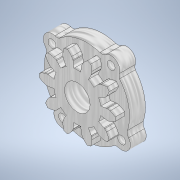
# Autodesk Inventor part: ｍ2歯数10ギア改二
Saved by Autodesk Inventor 2020.2 (Build 242310000, 310)
## iProperties
Created: 2019-11-09
Part Number: ｍ2歯数10ギア改二
Material: アルミニウム 7075
Document SubType Name: Modeling
Designer: aoyam
Density: 2.81 g/cm^3
Appearance: サテン - ブラシ仕上げ 重厚
Author: aoyam
Autodesk Inventor part; units mm, degrees
ref_plane "YZ Plane" through (0, 0, 0) normal (1, 0, 0) x (0, 1, 0)
ref_plane "XZ Plane" through (0, 0, 0) normal (0, 1, 0) x (-1, 0, 0)
ref_plane "XY Plane" through (0, 0, 0) normal (0, 0, 1) x (1, 0, 0)
sketch "スケッチ1" plane through (0, 0, 0) normal (0, 0, 1) x (1, 0, 0)
  arc A0 (-6.7711, 4.8044) -> (-6.8414, 4.5719) centre (-5.6655, 4.3429) ccw
  arc A1 (-6.3619, 5.5344) -> (-6.7711, 4.8044) centre (-3.6713, 3.5464) ccw
  arc A2 (-5.0279, 6.8503) -> (-6.3619, 5.5344) centre (-1.5449, 1.9856) ccw
  arc A3 (-9.5045, 4.5719) -> (-9.5748, 4.8044) centre (-10.6804, 4.3429) ccw
  arc A4 (-9.5748, 4.8044) -> (-9.984, 5.5344) centre (-12.6746, 3.5464) ccw
  arc A5 (-9.984, 5.5344) -> (-11.318, 6.8503) centre (-14.801, 1.9856) ccw
  arc A6 (-7.1102, 2.6941) -> (-9.2357, 2.6941) centre (-8.1729, -4.7302) ccw
  arc A7 (-11.318, 6.8503) -> (-12.4354, 6.4873) centre (-8.1729, -4.7302) ccw
  line L0 (-7.1102, 2.6941) -> (-6.8414, 4.5719)
  line L1 (-9.2357, 2.6941) -> (-9.5045, 4.5719)
  line L2 (-22.1729, -4.7302) -> (5.8271, -4.7302)
  line L3 (-8.1729, -18.7302) -> (-8.1729, 9.2698)
  arc A8 (-11.6771, 1.9009) -> (-13.3966, 0.6516) centre (-8.1729, -4.7302) ccw
  line L4 (-11.6771, 1.9009) -> (-12.5634, 3.578)
  line L5 (-13.3966, 0.6516) -> (-14.7178, 2.0127)
  arc A9 (-14.7178, 2.0127) -> (-14.9114, 2.1595) centre (-15.5346, 1.1363) ccw
  arc A10 (-12.4354, 6.4873) -> (-12.7411, 4.6385) centre (-6.7582, 4.5989) ccw
  arc A11 (-14.9114, 2.1595) -> (-15.6715, 2.5095) centre (-16.6797, -0.6803) ccw
  arc A12 (-15.6715, 2.5095) -> (-17.5242, 2.7901) centre (-17.4826, -3.1929) ccw
  arc A13 (-17.5242, 2.7901) -> (-18.2148, 1.8395) centre (-8.1729, -4.7302) ccw
  arc A14 (-12.6431, 3.8075) -> (-12.5634, 3.578) centre (-11.4774, 4.084) ccw
  arc A15 (-12.7411, 4.6385) -> (-12.6431, 3.8075) centre (-9.3959, 4.6117) ccw
  arc A16 (-14.9055, -1.4252) -> (-15.5623, -3.4467) centre (-8.1729, -4.7302) ccw
  line L6 (-14.9055, -1.4252) -> (-16.6083, -0.5893)
  line L7 (-15.5623, -3.4467) -> (-17.4312, -3.122)
  arc A17 (-17.4312, -3.122) -> (-17.6741, -3.1171) centre (-17.5768, -4.3112) ccw
  arc A18 (-18.2148, 1.8395) -> (-17.3755, 0.1642) centre (-12.5119, 3.6488) ccw
  arc A19 (-17.6741, -3.1171) -> (-18.4948, -3.2807) centre (-17.4355, -6.4539) ccw
  arc A20 (-18.4948, -3.2807) -> (-20.1586, -4.1427) centre (-16.6083, -8.9586) ccw
  arc A21 (-20.1586, -4.1427) -> (-20.1586, -5.3177) centre (-8.1729, -4.7302) ccw
  arc A22 (-16.8077, -0.4506) -> (-16.6083, -0.5893) centre (-16.0272, 0.4583) ccw
  arc A23 (-17.3755, 0.1642) -> (-16.8077, -0.4506) centre (-14.6534, 2.1087) ccw
  arc A24 (-15.5623, -6.0137) -> (-14.9055, -8.0351) centre (-8.1729, -4.7302) ccw
  line L8 (-15.5623, -6.0137) -> (-17.4312, -6.3384)
  line L9 (-14.9055, -8.0351) -> (-16.6083, -8.871)
  arc A25 (-16.6083, -8.871) -> (-16.8077, -9.0098) centre (-16.0272, -9.9187) ccw
  arc A26 (-20.1586, -5.3177) -> (-18.4948, -6.1797) centre (-16.6083, -0.5018) ccw
  arc A27 (-16.8077, -9.0098) -> (-17.3755, -9.6246) centre (-14.6534, -11.5691) ccw
  arc A28 (-17.3755, -9.6246) -> (-18.2148, -11.2999) centre (-12.5119, -13.1092) ccw
  arc A29 (-18.2148, -11.2999) -> (-17.5242, -12.2504) centre (-8.1729, -4.7302) ccw
  arc A30 (-17.6741, -6.3433) -> (-17.4312, -6.3384) centre (-17.5768, -5.1492) ccw
  arc A31 (-18.4948, -6.1797) -> (-17.6741, -6.3433) centre (-17.4355, -3.0065) ccw
  arc A32 (-13.3966, -10.1119) -> (-11.6771, -11.3612) centre (-8.1729, -4.7302) ccw
  line L10 (-13.3966, -10.1119) -> (-14.7178, -11.4731)
  line L11 (-11.6771, -11.3612) -> (-12.5634, -13.0384)
  arc A33 (-12.5634, -13.0384) -> (-12.6431, -13.2679) centre (-11.4774, -13.5443) ccw
  arc A34 (-17.5242, -12.2504) -> (-15.6715, -11.9699) centre (-17.4826, -6.2675) ccw
  arc A35 (-12.6431, -13.2679) -> (-12.7411, -14.0989) centre (-9.3959, -14.0721) ccw
  arc A36 (-12.7411, -14.0989) -> (-12.4354, -15.9476) centre (-6.7582, -14.0593) ccw
  arc A37 (-12.4354, -15.9476) -> (-11.318, -16.3107) centre (-8.1729, -4.7302) ccw
  arc A38 (-14.9114, -11.6198) -> (-14.7178, -11.4731) centre (-15.5346, -10.5967) ccw
  arc A39 (-15.6715, -11.9699) -> (-14.9114, -11.6198) centre (-16.6797, -8.7801) ccw
  arc A40 (-9.2357, -12.1545) -> (-7.1102, -12.1545) centre (-8.1729, -4.7302) ccw
  line L12 (-9.2357, -12.1545) -> (-9.5045, -14.0323)
  line L13 (-7.1102, -12.1545) -> (-6.8414, -14.0323)
  arc A41 (-6.8414, -14.0323) -> (-6.7711, -14.2648) centre (-5.6655, -13.8033) ccw
  arc A42 (-11.318, -16.3107) -> (-9.984, -14.9948) centre (-14.801, -11.446) ccw
  arc A43 (-6.7711, -14.2648) -> (-6.3619, -14.9948) centre (-3.6713, -13.0068) ccw
  arc A44 (-6.3619, -14.9948) -> (-5.0279, -16.3107) centre (-1.5449, -11.446) ccw
  arc A45 (-5.0279, -16.3107) -> (-3.9105, -15.9476) centre (-8.1729, -4.7302) ccw
  arc A46 (-9.5748, -14.2648) -> (-9.5045, -14.0323) centre (-10.6804, -13.8033) ccw
  arc A47 (-9.984, -14.9948) -> (-9.5748, -14.2648) centre (-12.6746, -13.0068) ccw
  arc A48 (-4.6688, -11.3612) -> (-2.9493, -10.1119) centre (-8.1729, -4.7302) ccw
  line L14 (-4.6688, -11.3612) -> (-3.7825, -13.0384)
  line L15 (-2.9493, -10.1119) -> (-1.6281, -11.4731)
  arc A49 (-1.6281, -11.4731) -> (-1.4345, -11.6198) centre (-0.8113, -10.5967) ccw
  arc A50 (-3.9105, -15.9476) -> (-3.6048, -14.0989) centre (-9.5877, -14.0593) ccw
  arc A51 (-1.4345, -11.6198) -> (-0.6744, -11.9699) centre (0.3338, -8.7801) ccw
  arc A52 (-0.6744, -11.9699) -> (1.1783, -12.2504) centre (1.1367, -6.2675) ccw
  arc A53 (1.1783, -12.2504) -> (1.8689, -11.2999) centre (-8.1729, -4.7302) ccw
  arc A54 (-3.7028, -13.2679) -> (-3.7825, -13.0384) centre (-4.8685, -13.5443) ccw
  arc A55 (-3.6048, -14.0989) -> (-3.7028, -13.2679) centre (-6.95, -14.0721) ccw
  arc A56 (-1.4404, -8.0351) -> (-0.7836, -6.0137) centre (-8.1729, -4.7302) ccw
  line L16 (-1.4404, -8.0351) -> (0.2624, -8.871)
  line L17 (-0.7836, -6.0137) -> (1.0853, -6.3384)
  arc A57 (1.0853, -6.3384) -> (1.3282, -6.3433) centre (1.2309, -5.1492) ccw
  arc A58 (1.8689, -11.2999) -> (1.0296, -9.6246) centre (-3.834, -13.1092) ccw
  arc A59 (1.3282, -6.3433) -> (2.1489, -6.1797) centre (1.0897, -3.0065) ccw
  arc A60 (2.1489, -6.1797) -> (3.8127, -5.3177) centre (0.2624, -0.5018) ccw
  arc A61 (3.8127, -5.3177) -> (3.8127, -4.1427) centre (-8.1729, -4.7302) ccw
  arc A62 (0.4618, -9.0098) -> (0.2624, -8.871) centre (-0.3187, -9.9187) ccw
  arc A63 (1.0296, -9.6246) -> (0.4618, -9.0098) centre (-1.6925, -11.5691) ccw
  arc A64 (-0.7836, -3.4467) -> (-1.4404, -1.4252) centre (-8.1729, -4.7302) ccw
  line L18 (-0.7836, -3.4467) -> (1.0853, -3.122)
  line L19 (-1.4404, -1.4252) -> (0.2624, -0.5893)
  arc A65 (0.2624, -0.5893) -> (0.4618, -0.4506) centre (-0.3187, 0.4583) ccw
  arc A66 (3.8127, -4.1427) -> (2.1489, -3.2807) centre (0.2624, -8.9586) ccw
  arc A67 (0.4618, -0.4506) -> (1.0296, 0.1642) centre (-1.6925, 2.1087) ccw
  arc A68 (1.0296, 0.1642) -> (1.8689, 1.8395) centre (-3.834, 3.6488) ccw
  arc A69 (1.8689, 1.8395) -> (1.1783, 2.7901) centre (-8.1729, -4.7302) ccw
  arc A70 (1.3282, -3.1171) -> (1.0853, -3.122) centre (1.2309, -4.3112) ccw
  arc A71 (2.1489, -3.2807) -> (1.3282, -3.1171) centre (1.0897, -6.4539) ccw
  arc A72 (-2.9493, 0.6516) -> (-4.6688, 1.9009) centre (-8.1729, -4.7302) ccw
  line L20 (-2.9493, 0.6516) -> (-1.6281, 2.0127)
  line L21 (-4.6688, 1.9009) -> (-3.7825, 3.578)
  arc A73 (-3.7825, 3.578) -> (-3.7028, 3.8075) centre (-4.8685, 4.084) ccw
  arc A74 (1.1783, 2.7901) -> (-0.6744, 2.5095) centre (1.1367, -3.1929) ccw
  arc A75 (-3.7028, 3.8075) -> (-3.6048, 4.6385) centre (-6.95, 4.6117) ccw
  arc A76 (-3.6048, 4.6385) -> (-3.9105, 6.4873) centre (-9.5877, 4.5989) ccw
  arc A77 (-3.9105, 6.4873) -> (-5.0279, 6.8503) centre (-8.1729, -4.7302) ccw
  arc A78 (-1.4345, 2.1595) -> (-1.6281, 2.0127) centre (-0.8113, 1.1363) ccw
  arc A79 (-0.6744, 2.5095) -> (-1.4345, 2.1595) centre (0.3338, -0.6803) ccw
  circle A80 centre (-8.1729, -4.7302) radius 2.5
  circle A81 centre (-8.1729, -4.7302) radius 4.025
  circle A82 centre (-8.1729, -4.7302) radius 12 construction
  circle A83 centre (-19.1875, 2.9441) radius 1.25
  arc A84 (-18.2949, 5.5452) -> (-21.3532, 1.2493) centre (-19.1875, 2.9441) ccw
  arc A85 (-18.2949, 5.5452) -> (-16.8738, 5.5919) centre (-17.6457, 7.4369) ccw
  arc A86 (-21.0243, -0.5958) -> (-21.3532, 1.2493) centre (-22.9282, 0.0167) ccw
  arc A87 (-18.4484, -14.8521) -> (-14.1525, -17.9104) centre (-15.8473, -15.7447) ccw
  circle A88 centre (-15.8473, -15.7447) radius 1.25
  arc A89 (-12.3074, -17.5815) -> (-14.1525, -17.9104) centre (-12.9199, -19.4854) ccw
  arc A90 (-18.4484, -14.8521) -> (-18.495, -13.431) centre (-20.3401, -14.2029) ccw
  arc A91 (1.949, -15.0056) -> (5.0073, -10.7097) centre (2.8416, -12.4045) ccw
  circle A92 centre (2.8416, -12.4045) radius 1.25
  arc A93 (4.6784, -8.8646) -> (5.0073, -10.7097) centre (6.5823, -9.4771) ccw
  arc A94 (1.949, -15.0056) -> (0.5279, -15.0523) centre (1.2998, -16.8973) ccw
  arc A95 (2.1025, 5.3917) -> (-2.1934, 8.45) centre (-0.4986, 6.2844) ccw
  circle A96 centre (-0.4986, 6.2844) radius 1.25
  arc A97 (-4.0385, 8.1211) -> (-2.1934, 8.45) centre (-3.426, 10.025) ccw
  arc A98 (2.1025, 5.3917) -> (2.1491, 3.9707) centre (3.9942, 4.7425) ccw
  arc A99 (-21.0243, -0.5958) -> (-18.495, -13.431) centre (-8.1729, -4.7302) ccw
  arc A100 (-12.3074, -17.5815) -> (0.5279, -15.0523) centre (-8.1729, -4.7302) ccw
  arc A101 (4.6784, -8.8646) -> (2.1491, 3.9707) centre (-8.1729, -4.7302) ccw
  arc A102 (-4.0385, 8.1211) -> (-16.8738, 5.5919) centre (-8.1729, -4.7302) ccw
  point P0 (0, 0)
  point P1 (-16.4019, 6.5961)
  point P2 (-21.4877, -0.4039)
  point P3 (-21.4877, -9.0564)
  point P4 (-16.4019, -16.0564)
  point P5 (-8.1729, -18.7302)
  point P6 (0.056, -16.0564)
  point P7 (5.1418, -9.0564)
  point P8 (5.1418, -0.4039)
  point P9 (0.056, 6.5961)
  point P10 (-18.4948, -3.2807)
  point P11 (-20.1586, -4.1427)
  point P12 (-20.1586, -5.3177)
  point P13 (-18.4948, -6.1797)
  point P14 (-17.6741, -6.3433)
  point P15 (-17.4312, -6.3384)
  point P16 (-15.5623, -6.0137)
  point P17 (-14.9055, -8.0351)
  point P18 (-16.8077, -9.0098)
  point P19 (-17.3755, -9.6246)
  point P20 (-18.2148, -11.2999)
  point P21 (-17.5242, -12.2504)
  point P22 (-15.6715, -11.9699)
  point P23 (-14.9114, -11.6198)
  point P24 (-13.3966, -10.1119)
  point P25 (-11.6771, -11.3612)
  point P26 (-12.5634, -13.0384)
  point P27 (-12.6431, -13.2679)
  point P28 (-12.7411, -14.0989)
  point P29 (-12.4354, -15.9476)
  point P30 (-11.318, -16.3107)
  point P31 (-9.984, -14.9948)
  point P32 (-9.5748, -14.2648)
  point P33 (-9.5045, -14.0323)
  point P34 (-9.2357, -12.1545)
  point P35 (-7.1102, -12.1545)
  point P36 (-6.7711, -14.2648)
  point P37 (-6.3619, -14.9948)
  point P38 (-5.0279, -16.3107)
  point P39 (-3.9105, -15.9476)
  point P40 (-3.6048, -14.0989)
  point P41 (-3.7028, -13.2679)
  point P42 (-3.7825, -13.0384)
  point P43 (-4.6688, -11.3612)
  point P44 (-2.9493, -10.1119)
  point P45 (-1.4345, -11.6198)
  point P46 (-0.6744, -11.9699)
  point P47 (1.1783, -12.2504)
  point P48 (1.8689, -11.2999)
  point P49 (1.0296, -9.6246)
  point P50 (0.4618, -9.0098)
  point P51 (0.2624, -8.871)
  point P52 (-1.4404, -8.0351)
  point P53 (-0.7836, -6.0137)
  point P54 (1.0853, -6.3384)
  point P55 (1.3282, -6.3433)
  point P56 (2.1489, -6.1797)
  point P57 (3.8127, -5.3177)
  point P58 (3.8127, -4.1427)
  point P59 (2.1489, -3.2807)
  point P60 (1.3282, -3.1171)
  point P61 (1.0853, -3.122)
  point P62 (-0.7836, -3.4467)
  point P63 (0.4618, -0.4506)
  point P64 (1.0296, 0.1642)
  point P65 (1.8689, 1.8395)
  point P66 (1.1783, 2.7901)
  point P67 (-0.6744, 2.5095)
  point P68 (-1.4345, 2.1595)
  point P69 (-1.6281, 2.0127)
  point P70 (-2.9493, 0.6516)
  point P71 (-4.6688, 1.9009)
  point P72 (-3.7825, 3.578)
  point P73 (-3.7028, 3.8075)
  point P74 (-3.6048, 4.6385)
  point P75 (-3.9105, 6.4873)
  point P76 (-5.0279, 6.8503)
  point P77 (-6.3619, 5.5344)
  point P78 (-6.7711, 4.8044)
  point P79 (-6.8414, 4.5719)
  point P80 (-7.1102, 2.6941)
  point P81 (-9.2357, 2.6941)
  point P82 (-9.5045, 4.5719)
  point P83 (-9.5748, 4.8044)
  point P84 (-9.984, 5.5344)
  point P85 (-11.318, 6.8503)
  point P86 (-12.4354, 6.4873)
  point P87 (-12.7411, 4.6385)
  point P88 (-12.6431, 3.8075)
  point P89 (-14.9114, 2.1595)
  point P90 (-15.6715, 2.5095)
  point P91 (-17.5242, 2.7901)
  point P92 (-18.2148, 1.8395)
  point P93 (-17.3755, 0.1642)
  point P94 (-16.8077, -0.4506)
  point P95 (-17.6741, -3.1171)
  point P96 (-12.4992, -18.045)
  point P97 (5.1418, -9.0564)
  point P98 (-3.8467, 8.5846)
  dimension "d2" = 360
  dimension "d6" = 5
  dimension "d7" = 1.525
  dimension "d8" = 8.05
  dimension "d10" = 2.5
  dimension "d11" = 1.5
  dimension "d12" = 2
  dimension "d15" = 360
  dimension "d19" = 13.4244
  constraints: 192 point on circle, 102 centre point, 44 end point, 4 coincident, 2 tangent, 1 equal radius, 1 midpoint, 441 other
  measures "d6" diameter of A80
  measures "d7" radial gap between concentric circles of A80 A81
  measures "d8" diameter of A81
  measures "d10" diameter of A83
  measures "d11" radial gap between concentric circles of A83 A84
  measures "d12" radius of A85
  measures "d19" distance of A6.centre A83.centre
extrude "押し出し1" add sketch "スケッチ1" along normal blind 3 contours A1 A2 A77 A76 A75 A73 L21 A72 L20 A78 A79 A74 A69 A68 A67 A65 L19 A64 L18 A70 A71 A66 A61 L2 A81 L3 A6 L0 A0 | L3 A81 L2 A21 A20 A19 A17 L7 A16 L6 A22 A23 A18 A13 A12 A11 A9 L5 A8 L4 A14 A15 A10 A7 A5 A4 A3 L1 A6 | L2 A61 A60 A59 A57 L17 A56 L16 A62 A63 A58 A53 A52 A51 A49 L15 A48 L14 A54 A55 A50 A45 A44 A43 A41 L13 A40 L3 A81 | A81 L3 A40 L12 A46 A47 A42 A37 A36 A35 A33 L11 A32 L10 A38 A39 A34 A29 A28 A27 A25 L9 A24 L8 A30 A31 A26 A21 L2
extrude "押し出し2" add sketch "スケッチ1" against normal blind 5 contours A1 A2 A77 A76 A75 A73 L21 A72 L20 A78 A79 A74 A69 A68 A67 A65 L19 A64 L18 A70 A71 A66 A61 L2 A81 L3 A6 L0 A0 | A0 L0 A6 L3 A102 A97 A95 A98 A101 L2 A61 A66 A71 A70 L18 A64 L19 A65 A67 A68 A69 A74 A79 A78 L20 A72 L21 A73 A75 A76 A77 A2 A1 | L3 A81 L2 A21 A20 A19 A17 L7 A16 L6 A22 A23 A18 A13 A12 A11 A9 L5 A8 L4 A14 A15 A10 A7 A5 A4 A3 L1 A6 | A6 L1 A3 A4 A5 A7 A10 A15 A14 L4 A8 L5 A9 A11 A12 A13 A18 A23 A22 L6 A16 L7 A17 A19 A20 A21 L2 A99 A86 A84 A85 A102 L3 | L2 A61 A60 A59 A57 L17 A56 L16 A62 A63 A58 A53 A52 A51 A49 L15 A48 L14 A54 A55 A50 A45 A44 A43 A41 L13 A40 L3 A81 | A81 L3 A40 L12 A46 A47 A42 A37 A36 A35 A33 L11 A32 L10 A38 A39 A34 A29 A28 A27 A25 L9 A24 L8 A30 A31 A26 A21 L2 | L2 A101 A93 A91 A94 A100 L3 A40 L13 A41 A43 A44 A45 A50 A55 A54 L14 A48 L15 A49 A51 A52 A53 A58 A63 A62 L16 A56 L17 A57 A59 A60 A61 | A21 A26 A31 A30 L8 A24 L9 A25 A27 A28 A29 A34 A39 A38 L10 A32 L11 A33 A35 A36 A37 A42 A47 A46 L12 A40 L3 A100 A89 A87 A90 A99 L2
